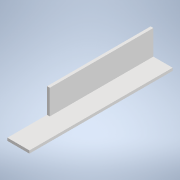
# Autodesk Inventor part: base
Saved by Autodesk Inventor 2020.2 (Build 242310000, 310)
## iProperties
Created: 2020-01-21
Part Number: base
Material: Generic
Document SubType Name: Modeling
Designer: robst
Density: 1 g/cm^3
Appearance: Default
Author: robst
Autodesk Inventor part; units mm, degrees
ref_plane "YZ Plane" through (0, 0, 0) normal (1, 0, 0) x (0, 1, 0)
ref_plane "XZ Plane" through (0, 0, 0) normal (0, 1, 0) x (-1, 0, 0)
ref_plane "XY Plane" through (0, 0, 0) normal (0, 0, 1) x (1, 0, 0)
sketch "Sketch1" plane through (0, 0, 0) normal (0, 0, 1) x (1, 0, 0)
  line L0 (0, 0) -> (50.8, 0)
  line L1 (0, 0) -> (0, 63.5)
  line L2 (0, 63.5) -> (6.35, 63.5)
  line L3 (6.35, 63.5) -> (6.35, 6.35)
  line L4 (6.35, 6.35) -> (50.8, 6.35)
  line L5 (50.8, 6.35) -> (50.8, 0)
  dimension "d0" = 50.8
  dimension "d1" = 63.5
  dimension "d2" = 6.35
  dimension "d3" = 6.35
  constraints: 12 end point, 4 perpendicular, 1 horizontal, 1 vertical
  measures "d0" distance of L0.start L0.end
  measures "d1" distance of L0.start L1.end
  measures "d2" distance of L1.end L2.end
  measures "d3" distance between parallel lines of L0 L4
extrude "Extrusion1" add sketch "Sketch1" along normal mid plane 330.2
sketch "Sketch3" plane through (6.35, 6.35, 165.1) normal (1, 0, 0) x (0, 0, -1)
  line L0 (0, 0) -> (0, 57.15) projected
  line L1 (330.2, 57.15) -> (0, 57.15) projected
  line L2 (0, 0) -> (91.44, 0)
  line L3 (91.44, 0) -> (91.44, 57.15)
  line L4 (91.44, 57.15) -> (0, 57.15)
  line L5 (0, 57.15) -> (0, 0)
  point P0 (165.1, -6.35)
  dimension "d6" = 91.44
  constraints: 8 end point, 2 parallel, 1 horizontal, 1 perpendicular, 1 point on line
  measures "d6" distance between parallel lines of L3 L0
extrude "Extrusion2" cut sketch "Sketch3" against normal through all
body "Solid1"
